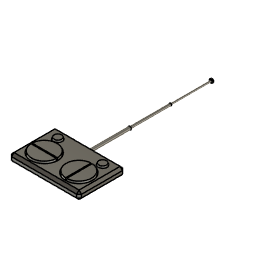
2024_10_14_BlackSubmarine v1 (Autodesk Fusion 360 design; units mm, degrees)
Autodesk Fusion 360 part; units mm, degrees
note: some values were not read from the file. Chosen so that the rebuilt part matches the saved one: which bodies a step acts on; which face or edge a step refers to. Set by a fixed rule: which sketch regions a step uses.
sketch "Sketch1" plane through (0, 0, 0) normal (0, 0, 1) x (1, 0, 0)
sketch "Sketch2" plane through (0, 0, 0) normal (0, 0, 1) x (1, 0, 0)
  circle A0 centre (-21.2754, -0.4884) radius 16.6728
  line L0 (-5.6386, 0.1758) -> (-36.9121, 0.1758)
  line L1 (-36.9121, -1.1525) -> (-5.6386, -1.1525)
  circle A1 centre (-27.4973, 22.4433) radius 4.6611
  circle A2 centre (-27.4973, 22.4433) radius 5.5101
  line L2 (42.9723, 34.457) -> (-42.9723, 34.457)
  line L3 (-42.9723, 34.457) -> (-42.9723, -34.457)
  line L4 (-42.9723, -34.457) -> (42.9723, -34.457)
  line L5 (42.9723, -34.457) -> (42.9723, 34.457)
  line L6 (42.9723, 34.457) -> (-42.9723, -34.457) construction
  line L7 (-42.9723, 34.457) -> (42.9723, -34.457) construction
  line L8 (-42.9723, -21.9671) -> (44.3013, -21.9671)
  circle A3 centre (-21.2754, -0.4884) radius 16.6728
  line L9 (0, 0) -> (0, 3.1008)
  circle A4 centre (21.2754, -0.4884) radius 16.6728
  line L10 (0, 0) -> (0, 3.1008)
  circle A5 centre (27.4973, 22.4433) radius 5.5101
  circle A6 centre (27.4973, 22.4433) radius 4.6611
  line L11 (-38.5579, 0.1758) -> (-37.9358, 0.1519) construction
  line L12 (-36.9147, 0.1126) -> (-5.6361, -1.0894) construction
  line L13 (-3.9928, 0.1758) -> (-4.6149, 0.1519) construction
  line L14 (-5.6361, 0.1126) -> (-36.9147, -1.0894) construction
  arc A7 (-5.6386, 0.1758) -> (-36.9121, 0.1758) centre (-21.2754, -0.4884) ccw
  arc A8 (-36.9121, -1.1525) -> (-5.6386, -1.1525) centre (-21.2754, -0.4884) ccw
  point P0 (-21.2754, -0.4884)
  constraint horizontal L0
  constraint parallel L0 L1
  constraint coincident P0 L13
  constraint coincident P0 L11
  constraint coincident P0 A0.centre
  constraint concentric A1 A2
  constraint horizontal L2
  constraint perpendicular L2 L3
  constraint parallel L2 L4
  constraint parallel L3 L5
  constraint coincident L6 L9.start
  constraint coincident L7 L9.start
  constraint coincident L9.start L10.start
  constraint coincident L3 L8.start
  constraint perpendicular L5 L8
  constraint vertical L9
  constraint symmetric A0 L9 A4
  constraint symmetric L10.start L9 origin
  constraint symmetric L10.end L9 L9.end
  constraint symmetric A1 L9 A6
  constraint symmetric A2 L9 A5
  constraint coincident L14.end A7
  constraint coincident L1.start A7
  constraint coincident A0 L11.end
  constraint collinear L11 L12
  constraint coincident A0 L13.end
  constraint collinear L13 L14
  constraint concentric A0 A7
  constraint concentric A7 A8
extrude "Extrude1" add sketch "Sketch2" against normal blind 10 contours A0 A3 | L0 A7 | L1 A8 | A1 | A2 | L2 L3 L5 L8 | A4 | A5 | A6 makes body 1
extrude "Extrude2" cut sketch "Sketch2" against normal blind 5 contours A0 A3 | L0 A7 | L1 A8 | A1 | A2 bodies 1
extrude "Extrude3" add sketch "Sketch2" along normal blind 2 and the other way blind 2 separate body contours L0 A7 | L1 A8 | A1 makes body 2 at (-25.3027, 5.0737, 2) makes body 3 at (-25.5153, -7.501, 2) makes body 4 at (-29.9267, 22.4155, 2)
extrude "Extrude4" cut sketch "Sketch2" against normal blind 5 contours A4 | A5 | A6 bodies 1
mirror "Mirror1" about plane through (0, 0, 0) normal (1, 0, 0) of bodies 4 2 3 makes body 5 at (25.3027, 5.0737, 2) makes body 6 at (25.5153, -7.501, 2) makes body 7 at (29.9267, 22.4155, 2)
move_body "Move1" bodies 5 6 to x (0, -1, 0) y (1, 0, 0) z (0, 0, 1) at (21.7637, 20.787, 0)
sketch "Sketch3" plane through (0, 0, 0) normal (0, 0, 1) x (1, 0, 0)
  line L0 (0, 33.2952) -> (-2, 33.2952)
  line L1 (-2, 33.2952) -> (-2, 83.2952)
  line L2 (-2, 83.2952) -> (0, 83.2952)
  line L3 (0, 83.2952) -> (0, 33.2952)
  line L4 (0, 83.2952) -> (-1.5, 83.2952)
  line L5 (-1.5, 83.2952) -> (-1.5, 133.2952)
  line L6 (-1.5, 133.2952) -> (0, 133.2952)
  line L7 (0, 133.2952) -> (0, 83.2952)
  line L8 (0, 133.2952) -> (-1, 133.2952)
  line L9 (-1, 133.2952) -> (-1, 183.2952)
  line L10 (-1, 183.2952) -> (0, 183.2952)
  line L11 (0, 183.2952) -> (0, 133.2952)
  line L12 (0, 183.2952) -> (-2.2, 183.2952)
  line L13 (-2.2, 183.2952) -> (-2.2, 184.2952)
  line L14 (-2.2, 184.2952) -> (0, 184.2952)
  line L15 (0, 184.2952) -> (0, 183.2952)
  dimension "d15" = 2
  dimension "d16" = 50
  dimension "d17" = 1.5
  dimension "d18" = 50
  dimension "d19" = 1
  dimension "d20" = 50
  dimension "d21" = 2.2
  dimension "d22" = 1
  constraint horizontal L0
  constraint vertical L1
  constraint horizontal L2
  constraint vertical L3
  constraint horizontal L4
  constraint vertical L5
  constraint horizontal L6
  constraint vertical L7
  constraint horizontal L8
  constraint vertical L9
  constraint horizontal L10
  constraint vertical L11
  constraint horizontal L12
  constraint vertical L13
  constraint horizontal L14
  constraint vertical L15
  measures "d15" distance of L0.start L0.end
  measures "d16" distance of L0.start L2.end
  measures "d17" distance of L2.end L4.end
  measures "d18" distance of L2.end L6.end
  measures "d19" distance of L6.end L8.end
  measures "d20" distance of L6.end L10.end
  measures "d21" distance of L10.end L12.end
  measures "d22" distance of L10.end L14.end
revolve "Revolve1" add sketch "Sketch3" angle 360 about axis through (0, 183.2952, 0) along (0, -1, 0) separate body contours L6 L8 L9 L10 L11 L12 | L10 L12 L13 L14 L15 makes body 8
revolve "Revolve2" add sketch "Sketch3" angle 360 about axis through (0, 133.2952, 0) along (0, -1, 0) separate body contours L2 L4 L5 L6 L7 L8 makes body 9
revolve "Revolve3" add sketch "Sketch3" angle 360 about axis through (0, 83.2952, 0) along (0, -1, 0) separate body contours L0 L1 L2 L3 L4 makes body 10
chamfer "Chamfer1" distance 3 angle 45 4 faces at (-42.9723, 15.649, -6.6667) (14.3241, 34.457, -3.3333) (-14.3241, -21.9671, -3.3333) (42.9723, -3.159, -6.6667) on bodies 1
move_body "Move2" bodies 10 8 9 to x (1, 0, 0) y (0, 1, 0) z (0, 0, 1) at (0, 0, -5)
named bodies: "BodyRC", "ForwardButton", "BackwardButton", "UpButton", "RightButton", "LeftButton", "DownButton", "Antenna3", "Antenna2", "Antenna1"
